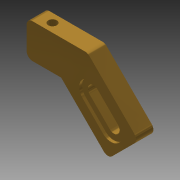
# Autodesk Inventor part: HW 7 Part 5
Saved by Autodesk Inventor 2015 (Build 190159000, 159)
## iProperties
Created: 2016-02-24
Part Number: HW 7 Part 5
Material: Brass, Soft Yellow
Document SubType Name: Modeling
Designer: Melissa
Density: 8.47 g/cm^3
Appearance: Brass - Satin
Mass: 4.95481e+07 g
Surface Area: 313151 cm^2
Volume: 5.84983e+06 cm^3
Author: Melissa
Autodesk Inventor part; units mm, degrees
ref_plane "YZ Plane" through (0, 0, 0) normal (1, 0, 0) x (0, 1, 0)
ref_plane "XZ Plane" through (0, 0, 0) normal (0, 1, 0) x (-1, 0, 0)
ref_plane "XY Plane" through (0, 0, 0) normal (0, 0, 1) x (1, 0, 0)
sketch "Sketch1" plane through (0, 0, 0) normal (0, 0, 1) x (1, 0, 0)
  line L0 (0, 254) -> (0, 1270)
  line L1 (254, 1524) -> (2588.8666, 1524)
  line L2 (2768.4717, 1449.6051) -> (4756.8922, -538.8154)
  line L3 (4756.8922, -898.0256) -> (3769.064, -1885.8538)
  line L4 (3409.8538, -1885.8538) -> (1524, 0)
  line L5 (1524, 0) -> (254, 0)
  arc A0 (254, 1524) -> (0, 1270) centre (254, 1270) ccw
  arc A1 (0, 254) -> (254, 0) centre (254, 254) ccw
  arc A2 (3409.8538, -1885.8538) -> (3769.064, -1885.8538) centre (3589.4589, -1706.2487) ccw
  arc A3 (4756.8922, -898.0256) -> (4756.8922, -538.8154) centre (4577.2871, -718.4205) ccw
  line L6 (2826.1371, 44.9013) -> (3724.1627, -853.1243) construction
  line L7 (3005.7423, 224.5064) -> (3903.7679, -673.5192)
  line L8 (3544.5576, -1032.7295) -> (2646.532, -134.7038)
  arc A4 (3005.7423, 224.5064) -> (2646.532, -134.7038) centre (2826.1371, 44.9013) ccw
  arc A5 (3544.5576, -1032.7295) -> (3903.7679, -673.5192) centre (3724.1627, -853.1243) ccw
  line L9 (2826.1371, 44.9013) -> (3724.1627, -853.1243) construction
  line L10 (2466.9269, -314.309) -> (3364.9525, -1212.3346)
  line L11 (4083.373, -493.9141) -> (3185.3474, 404.1115)
  arc A6 (3185.3474, 404.1115) -> (2466.9269, -314.309) centre (2826.1371, 44.9013) ccw
  arc A7 (3364.9525, -1212.3346) -> (4083.373, -493.9141) centre (3724.1627, -853.1243) ccw
  arc A8 (2768.4717, 1449.6051) -> (2588.8666, 1524) centre (2588.8666, 1270) ccw
  point P0 (0, 0)
  point P1 (0, 1524)
  point P2 (2694.0768, 1524)
  point P3 (4936.4973, -718.4205)
  point P4 (3589.4589, -2065.4589)
  point P5 (3275.1499, -404.1115)
  point P6 (3275.1499, -404.1115)
  dimension "d3" = 1524
  dimension "d4" = 1524
  dimension "d5" = 45
  dimension "d6" = 1905
  dimension "d9" = 2921
  dimension "d10" = 254
  dimension "d11" = 1270
  dimension "d12" = 508
  dimension "d13" = 762
  dimension "d14" = 952.5
  dimension "d15" = 254
  dimension "d26" = 254
  constraints: 28 end point, 18 point on circle, 18 tangent, 10 point on line, 9 centre point, 5 parallel, 3 equal radius, 2 midpoint, 2 perpendicular, 1 collinear, 1 vertical
  measures "d3" distance of point (0, 0) point (0, 1524)
  measures "d4" distance of L4.end point (0, 0)
  measures "d5" angle of L1 L2
  measures "d6" distance of point (4936.497, -718.42) point (3589.459, -2065.459)
  measures "d9" distance of point (3589.459, -2065.459) L4.end
  measures "d10" radius of A0
  measures "d11" distance of L6.end L6.start
  measures "d12" distance between parallel lines of L7 L8
  measures "d13" distance from line of L3 L6.end
  measures "d14" distance from line of L4 L6.end
  measures "d15" distance between parallel lines of L11 L7
  measures "d26" radius of A8
extrude "Extrusion1" add sketch "Sketch1" against normal blind 762 contours L0 A0 L1 A8 L2 A3 L3 A2 L4 L5 A1 | A6 L11 A7 L10
extrude "Extrusion2" cut sketch "Sketch1" against normal blind 127 contours A6 L11 A7 L10
sketch "Sketch2" plane through (254, 0, 0) normal (0, -1, 0) x (1, 0, 0)
  circle A0 centre (508, -381) radius 190.5
  line L0 (1270, -762) -> (0, -762) projected
  line L1 (0, 0) -> (0, -762) projected
  point P0 (-254, 0)
  dimension "d20" = 381
  dimension "d21" = 381
  dimension "d23" = 762
  constraints: 1 centre point
  measures "d20" diameter of A0
  measures "d21" distance from line of L0 A0.centre
  measures "d23" horizontal distance of point (-254, 0) A0.centre
extrude "Extrusion3" cut sketch "Sketch2" against normal through all
body "Solid1"
